Drawer Reinforcement (Autodesk Fusion 360 design; units mm, degrees)
Autodesk Fusion 360 part; units mm, degrees
sketch "Sketch1" plane through (0, 0, 0) normal (0, 1, 0) x (1, 0, 0)
  line L0 (0, 0) -> (0, -76.2)
  line L1 (0, 0) -> (76.2, 0)
  line L2 (5, -5) -> (5, -76.2)
  line L3 (5, -5) -> (76.2, -5)
  line L4 (76.2, -5) -> (76.2, 0)
  line L5 (0, -76.2) -> (5, -76.2)
  dimension "d1" = 76.2
  constraint coincident L0.start L1.start
  constraint vertical L0
  constraint perpendicular L0 L1
  constraint equal L0 L1
  constraint perpendicular L1 L4
  constraint perpendicular L2 L5
  constraint coincident L2.start L3.start
  measures "d1" distance of L0.start L1.end
extrude "Extrude1" add sketch "Sketch1" along normal blind 15 makes body 1
ref_plane "WorkPlane1" through (2, 7.5, 40.6) normal (1, 0, 0) x (0, 0, -1)
sketch "Sketch4" plane through (2, 0, 0) normal (1, 0, 0) x (0, 1, 0)
  line L0 (0, 76.2) -> (0, 5)
  line L1 (15, 5) -> (15, 76.2)
  line L2 (15, 76.2) -> (0, 76.2)
  line L3 (0, 40.6) -> (15, 40.6) construction
  line L4 (7.5, 76.2) -> (7.5, 40.6) construction
  line L5 (7.5, 40.6) -> (7.5, 35.6) construction
  circle A0 centre (7.5, 58.4) radius 2
  circle A1 centre (7.5, 38.1) radius 2
  line L6 (0, 5) -> (15, 5)
  dimension "d17" = 4
  dimension "d30" = 4
  constraint midpoint L0 L3.start
  constraint midpoint L1 L3.end
  constraint midpoint L2 L4.start
  constraint midpoint L3 L4.end
  constraint midpoint L4 A0.centre
  constraint midpoint L5 A1.centre
  measures "d17" diameter of A0
  measures "d30" diameter of A1
extrude "Extrude4" cut sketch "Sketch4" against normal up to surface (2 mm away) contours A0 | A1 bodies 1
sketch "Sketch5" plane through (5, 0, 0) normal (1, 0, 0) x (0, 1, 0)
  line L0 (0, 76.2) -> (0, 5)
  line L1 (15, 5) -> (15, 76.2)
  line L2 (15, 76.2) -> (0, 76.2)
  circle A0 centre (7.5, 58.4) radius 2
  circle A1 centre (7.5, 58.4) radius 4
  circle A2 centre (7.5, 38.1) radius 4
  circle A3 centre (7.5, 38.1) radius 2
  line L3 (0, 5) -> (15, 5)
  dimension "d21" = 8
  dimension "d23" = 8
  constraint concentric A0 A1
  constraint concentric A2 A3
  measures "d21" diameter of A1
  measures "d23" diameter of A2
loft "Loft1" cut profiles "Sketch4", "Sketch5" section 1 contours A0 section 2 contours A0 | A1 bodies 1
loft "Loft3" cut profiles "Sketch5", "Sketch4" section 1 contours A2 | A3 section 2 contours A1 bodies 1
ref_plane "WorkPlane2" through (40.6, 7.5, 2) normal (0, 0, 1) x (1, 0, 0)
sketch "Sketch6" plane through (0, 0, 2) normal (0, 0, 1) x (1, 0, 0)
  line L0 (5, 0) -> (76.2, 0)
  line L1 (76.2, 0) -> (76.2, 15)
  line L2 (76.2, 15) -> (5, 15)
  line L3 (40.6, 15) -> (40.6, 0) construction
  line L4 (35.6, 7.5) -> (40.6, 7.5) construction
  line L5 (40.6, 7.5) -> (76.2, 7.5) construction
  circle A0 centre (58.4, 7.5) radius 2
  circle A1 centre (38.1, 7.5) radius 2
  line L6 (5, 15) -> (5, 0)
  dimension "d25" = 4
  dimension "d29" = 4
  constraint midpoint L2 L3.start
  constraint midpoint L0 L3.end
  constraint midpoint L3 L4.end
  constraint midpoint L1 L5.end
  constraint midpoint L5 A0.centre
  constraint midpoint L4 A1.centre
  measures "d25" diameter of A0
  measures "d29" diameter of A1
extrude "Extrude5" cut sketch "Sketch6" against normal up to surface (2 mm away) contours A0 | A1 bodies 1
sketch "Sketch7" plane through (0, 0, 5) normal (0, 0, 1) x (-1, 0, 0)
  line L0 (-5, 0) -> (-76.2, 0)
  line L1 (-76.2, 0) -> (-76.2, -15)
  line L2 (-76.2, -15) -> (-5, -15)
  circle A0 centre (-38.1, -7.5) radius 2
  circle A1 centre (-58.4, -7.5) radius 2
  circle A2 centre (-38.1, -7.5) radius 4
  circle A3 centre (-58.4, -7.5) radius 4
  line L3 (-5, -15) -> (-5, 0)
  dimension "d31" = 8
  dimension "d32" = 8
  constraint concentric A0 A2
  constraint concentric A1 A3
  measures "d31" diameter of A2
  measures "d32" diameter of A3
loft "Loft4" cut profiles "Sketch7", "Sketch6" section 1 contours A0 | A2 section 2 contours A1 bodies 1
loft "Loft5" cut profiles "Sketch7", "Sketch6" section 1 contours A1 | A3 section 2 contours A0 bodies 1
copy_body "CopyPasteBodies1" bodies 1 makes body 2
sketch "Sketch8" plane through (0, 0, 0) normal (0, -1, 0) x (1, 0, 0)
  line L0 (0, 76.2) -> (0, 0)
  line L1 (0, 0) -> (76.2, 0)
  line L2 (76.2, 0) -> (76.2, 5)
  line L3 (76.2, 5) -> (5, 5)
  line L4 (5, 5) -> (5, 76.2)
  line L5 (5, 76.2) -> (0, 76.2)
  line L6 (5, 76.2) -> (76.2, 5)
  line L7 (5, 62.0579) -> (62.0579, 5)
  dimension "d55" = 10
  constraint coincident L4.end L5.start
  constraint coincident L2.end L3.start
  constraint coincident L4 L7.start
  constraint coincident L3 L7.end
  constraint parallel L6 L7
  measures "d55" distance of L6 L7
extrude "Extrude6" add sketch "Sketch8" along normal blind 1.5 contours L0 L1 L2 L3 L4 L5 | L3 L4 L6 L7 bodies 1
sketch "Sketch9" plane through (0, 15, 0) normal (0, 1, 0) x (-1, 0, 0)
  line L0 (0, 0) -> (0, 76.2)
  line L1 (0, 76.2) -> (-5, 76.2)
  line L2 (-5, 76.2) -> (-5, 5)
  line L3 (-5, 5) -> (-76.2, 5)
  line L4 (-76.2, 5) -> (-76.2, 0)
  line L5 (-76.2, 0) -> (0, 0)
  line L6 (-5, 76.2) -> (-76.2, 5)
  line L7 (-62.0579, 5) -> (-5, 62.0579)
  dimension "d56" = 10
  constraint coincident L1.end L2.start
  constraint coincident L3.end L4.start
  constraint coincident L3 L7.start
  constraint coincident L2 L7.end
  constraint parallel L6 L7
  measures "d56" distance of L6 L7
extrude "Extrude7" add sketch "Sketch9" along normal blind 1.5 contours L0 L1 L2 L3 L4 L5 | L2 L3 L6 L7 bodies 2
fillet "Fillet4" radius 1 18 edges at (5, 7.5, 76.2) (0, 8.25, 76.2) (2.5, 0, 76.2) (2.5, 16.5, 76.2) (5, 15.75, 76.2) (0, 16.5, 38.1) (0, 0, 38.1) (5, 0, 40.6) (38.1, 0, 0) (76.2, 8.25, 0) (40.6, 0, 5) (76.2, 7.5, 5) (76.2, 0, 2.5) (76.2, 16.5, 2.5) (76.2, 15.75, 5) (38.1, 16.5, 0) (33.5289, 16.5, 5) (5, 16.5, 33.5289) on bodies 2
fillet "Fillet5" radius 0.5 12 edges at (4.2929, 15, 76.2) (4.9685, 15, 76.1239) (40.6, 15, 40.6) (76.1239, 15, 4.9685) (76.2, 15, 4.2929) (4.9685, 15.8827, 76.1239) (5.6173, 16.4239, 75.5827) (40.6, 16.5, 40.6) (75.5827, 16.4239, 5.6173) (76.1239, 15.8827, 4.9685) (33.5289, 16.5, 33.5289) (33.5289, 15, 33.5289) on bodies 2
fillet "Fillet6" radius 1 6 edges at (5, 15, 40.6) (0, 15, 38.1) (38.1, -1.5, 0) (0, -1.5, 38.1) (5, -1.5, 33.5289) (33.5289, -1.5, 5) 3 faces at (1.6667, 4.5, 76.2) (76.2, 4.5, 1.6667) (1.6667, 15, 27.0667) on bodies 1
fillet "Fillet7" [suppressed]
equation "d17 = Thread_Diameter"
equation "d21 = Head_Diameter"
equation "d23 = Head_Diameter"
equation "d25 = Thread_Diameter"
equation "Thread_Diameter = 4 mm"
equation "Head_Diameter = 8 mm"
equation "d29 = Thread_Diameter"
equation "d30 = Thread_Diameter"
equation "d31 = Head_Diameter"
equation "d32 = Head_Diameter"
